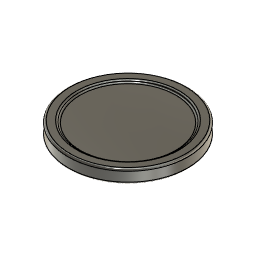
Puck v3 (Autodesk Fusion 360 design; units mm, degrees)
Autodesk Fusion 360 part; units mm, degrees
note: some values were not read from the file. Chosen so that the rebuilt part matches the saved one: which pieces of a blend or face edit are solid.
sketch "Skizze1" plane through (0, 0, 0) normal (0, 0, 1) x (1, 0, 0)
  circle A0 centre (0, 0) radius 31.5
  dimension "d1" = 63
  constraint coincident A0.centre origin
  measures "d1" diameter of A0
extrude "Extrusion1" add sketch "Skizze1" along normal blind 7
sketch "Skizze2" plane through (0, 0, 7) normal (0, 0, 1) x (-1, 0, 0)
  circle A0 centre (0, 0) radius 26
  circle A1 centre (0, 0) radius 31.5
  dimension "d5" = 52
  constraint coincident A0.centre A1.centre
  measures "d5" diameter of A0
extrude "Extrusion2" cut sketch "Skizze2" against normal blind 1.1 contours A0
sketch "Skizze3" plane through (0, 0, 0) normal (0, 0, -1) x (1, 0, 0)
  circle A0 centre (0, 0) radius 26
  circle A1 centre (0, 0) radius 31.5
  dimension "d8" = 52
  constraint coincident A0.centre A1.centre
  measures "d8" diameter of A0
extrude "Extrusion3" cut sketch "Skizze3" against normal blind 1.1 contours A0
fillet "Abrundung1" radius 1 5 edges at (-29.3683, -11.3909, 7) (-29.3683, -11.3909, 0) (24.2405, -9.402, 7) (-24.2405, -9.402, 1.1) (-24.2405, -9.402, 0) 1 faces at (-4.3333, -7.5056, 5.9)
